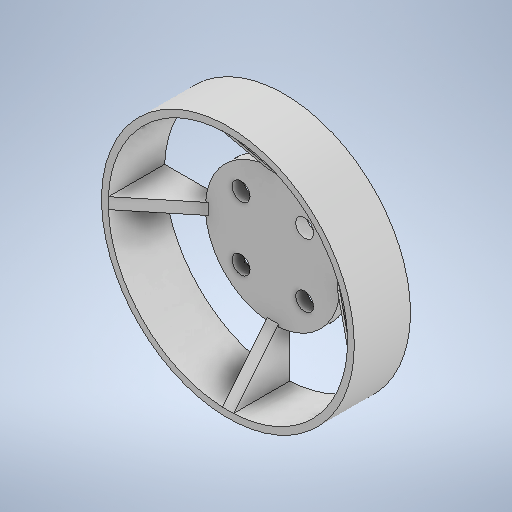
# Autodesk Inventor part: Wheel-D45A
Saved by Autodesk Inventor 2025.3 (Build 293356000, 356)
## iProperties
Created: 2025-07-18
Part Number: Wheel-D45A
Material: 一般
Document SubType Name: Modeling
Designer: yamashita1
Density: 1 g/cm^3
Appearance: 既定
Author: yamashita1
Autodesk Inventor part; units mm, degrees
ref_plane "YZ Plane" through (0, 0, 0) normal (1, 0, 0) x (0, 1, 0)
ref_plane "XZ Plane" through (0, 0, 0) normal (0, 1, 0) x (-1, 0, 0)
ref_plane "XY Plane" through (0, 0, 0) normal (0, 0, 1) x (1, 0, 0)
sketch "スケッチ1" plane through (0, 0, 0) normal (0, 0, 1) x (1, 0, 0)
  circle A0 centre (0, 0) radius 12
  dimension "HUB_DIA" = 24
  constraints: 1 centre point, 1 coincident
  measures "HUB_DIA" diameter of A0
extrude "ハブ" add sketch "スケッチ1" along normal blind 2
sketch "スケッチ2" plane through (0, 0, 0) normal (0, 0, 1) x (1, 0, 0)
  circle A0 centre (0, 0) radius 22.5
  circle A1 centre (0, 0) radius 21.3
  dimension "DIA" = 45
  dimension "RIM_THIN" = 1.2
  constraints: 2 centre point, 2 coincident
  measures "DIA" diameter of A0
  measures "RIM_THIN" radial gap between concentric circles of A0 A1
extrude "リム" add sketch "スケッチ2" along normal blind 10
sketch "スケッチ5" plane through (0, 0, 0) normal (1, 0, 0) x (0, 1, 0)
  line L0 (21.3, 10) -> (21.3, 0) projected
  line L1 (21.3, 10) -> (21.3, 0)
  line L2 (21.3, 0) -> (11.5, 0)
  line L3 (22.5, 0) -> (-22.5, 0) projected
  line L4 (11.5, 0) -> (11.5, 2)
  line L5 (11.5, 2) -> (21.3, 10)
  line L6 (12, 2) -> (-12, 2) projected
  point P0 (0, 0)
  point P1 (0, 0)
  dimension "d10" = 11.5
  constraints: 8 end point, 4 point on line, 1 midpoint, 1 vertical
  measures "d10" distance from line of point (0, 0) L4
extrude "スポーク" add sketch "スケッチ5" along normal mid plane 2
pattern_circular "円形状パターン1" count 4 over 360 about axis through (0, 0, -10) along (0, 0, 1) of "スポーク"
sketch "スケッチ6" plane through (0, 0, 2) normal (0, 0, 1) x (1, 0, 0)
  circle A0 centre (0, 0) radius 8 construction
  line L0 (-13.4189, -13.4189) -> (13.4189, 13.4189) construction
  line L1 (-15.0493, 15.0493) -> (15.0493, -15.0493) construction
  line L2 (-16.6434, 0) -> (16.6434, 0) construction
  point P0 (5.6569, 5.6569)
  point P1 (-5.6569, 5.6569)
  point P2 (-5.6569, -5.6569)
  point P3 (5.6569, -5.6569)
  dimension "d16" = 16
  dimension "d17" = 45
  dimension "d18" = 45
  constraints: 6 end point, 4 point on circle, 4 point on line, 3 midpoint, 2 coincident, 1 centre point, 1 horizontal
  measures "d16" diameter of A0
  measures "d17" angle of L0 L2
  measures "d18" angle of L2 L1
hole "フランジ取付穴" at (5.6569, 5.6569, 2) at (-5.6569, 5.6569, 2) at (-5.6569, -5.6569, 2) at (5.6569, -5.6569, 2) direction (0, 0, -1) diameter 3.2 end through all
sketch "スケッチ8" plane through (0, 0, 0) normal (0, 0, -1) x (-1, 0, 0)
  circle A0 centre (5.6569, 5.6569) radius 1.6 construction
  line L0 (5.6569, 5.6569) -> (10.4286, 10.4286) construction
  line L1 (5.6569, 5.6569) -> (12.4051, 5.6569) construction
  line L2 (5.7276, 5.5861) -> (5.5861, 5.7276)
  line L3 (5.5861, 5.7276) -> (11.243, 11.3844)
  line L4 (11.243, 11.3844) -> (11.3844, 11.243)
  line L5 (11.3844, 11.243) -> (5.7276, 5.5861)
  point P0 (0, 0)
  dimension "d32" = 45
  dimension "d33" = 8
  dimension "d34" = 0.2
  constraints: 12 end point, 3 parallel, 1 equal length, 1 horizontal, 1 midpoint, 1 perpendicular
  measures "d32" angle of L1 L0
  measures "d33" distance of L4.end L2.start
  measures "d34" distance of L3.end L4.end
extrude "1層目をきれいに出力する溝" cut sketch "スケッチ8" against normal blind 0.2
pattern_circular "円形状パターン2" count 4 over 360 about axis through (0, 0, -10) along (0, 0, 1) of "1層目をきれいに出力する溝"
equation "\"d18\" = d17"
